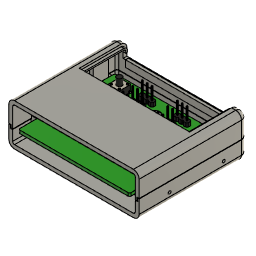
openC64case v22 (Autodesk Fusion 360 design; units mm, degrees)
Autodesk Fusion 360 part; units mm, degrees
(part 1 of 2)
sketch "Skizze1" plane through (0, 0, 0) normal (0, 0, 1) x (1, 0, 0)
  line L0 (44.1492, 35.54) -> (43.8162, 36.0162)
  line L1 (41.7212, 35.54) -> (41.7212, 36.54)
  line L2 (44.1492, 36.3495) -> (44.1492, 36.2067)
  line L3 (44.9592, 36.54) -> (45.0542, 36.4924)
  line L4 (42.5302, 36.54) -> (43.1972, 35.54)
  line L5 (42.5382, 48.2051) -> (42.4902, 48.3956)
  line L6 (43.5782, 35.54) -> (43.5782, 36.54)
  line L7 (42.4902, 48.7289) -> (42.5382, 48.9194)
  line L8 (43.5782, 36.54) -> (43.9592, 36.54)
  line L9 (42.1972, 35.54) -> (41.7212, 35.54)
  line L10 (44.7682, 36.54) -> (44.9592, 36.54)
  line L11 (43.1972, 36.54) -> (42.5302, 35.54)
  line L12 (45.6262, 36.54) -> (45.9592, 35.8257)
  line L13 (44.0542, 36.0638) -> (43.9592, 36.0162)
  line L14 (42.6332, 48.1098) -> (42.5382, 48.2051)
  line L15 (45.0542, 35.5876) -> (44.9592, 35.54)
  line L16 (42.2922, 41.0613) -> (42.1022, 41.0613)
  line L17 (44.5782, 36.3972) -> (44.6732, 36.4924)
  line L18 (45.1492, 35.6829) -> (45.0542, 35.5876)
  line L19 (45.1972, 35.8734) -> (45.1492, 35.6829)
  line L20 (42.6332, 49.0146) -> (42.7292, 49.0622)
  line L21 (44.9592, 35.54) -> (44.7682, 35.54)
  line L22 (45.0542, 36.4924) -> (45.1492, 36.3972)
  line L23 (43.9592, 36.54) -> (44.0542, 36.4924)
  line L24 (44.1492, 36.2067) -> (44.1022, 36.1114)
  line L25 (42.1492, 41.6327) -> (42.0062, 41.6327)
  line L26 (44.5782, 35.6829) -> (44.5302, 35.8734)
  line L27 (42.5382, 48.9194) -> (42.6332, 49.0146)
  line L28 (41.7212, 36.54) -> (42.1972, 36.54)
  line L29 (43.9592, 36.0162) -> (43.5782, 36.0162)
  line L30 (44.6732, 35.5876) -> (44.5782, 35.6829)
  line L31 (42.5782, 40.6327) -> (42.9112, 41.6327)
  line L32 (43.5782, 41.6327) -> (43.9112, 40.9184)
  line L33 (44.1022, 36.1114) -> (44.0542, 36.0638)
  line L34 (44.0542, 36.4924) -> (44.1022, 36.4448)
  line L35 (41.6732, 41.0613) -> (41.7212, 40.8708)
  line L36 (42.6732, 40.9184) -> (43.1492, 40.9184)
  line L37 (45.6262, 35.54) -> (45.6262, 36.54)
  line L38 (45.1492, 36.3972) -> (45.1972, 36.2067)
  line L39 (41.7212, 36.0638) -> (42.0542, 36.0638)
  line L40 (44.1972, 27.6866) -> (14.7332, 27.6866)
  line L41 (28.1952, 27.6866) -> (28.1952, 17.5266)
  line L42 (42.0062, 41.6327) -> (41.8642, 41.5851)
  line L43 (48.2612, 15.4946) -> (48.2612, 29.7186)
  line L44 (8.1452, 19.1706) -> (8.1452, 26.1706)
  line L45 (11.6852, 21.3366) -> (10.6692, 21.3366)
  line L46 (57.6592, 0.0006) -> (0.7632, 0.0006)
  line L47 (47.2452, 31.4966) -> (47.2452, 13.7166)
  line L48 (44.7212, 40.6327) -> (44.7212, 41.6327)
  line L49 (11.6852, 23.8766) -> (11.6852, 21.3366)
  line L50 (43.9112, 40.9184) -> (44.2452, 41.6327)
  line L51 (41.8642, 40.6803) -> (42.0062, 40.6327)
  line L52 (41.7212, 41.3946) -> (41.6732, 41.2041)
  line L53 (11.6852, 13.7166) -> (11.6852, 31.4966)
  line L54 (46.2922, 36.54) -> (46.2922, 35.54)
  line L55 (48.2612, 29.7186) -> (10.6692, 29.7186)
  line L56 (42.2452, 41.5851) -> (42.1492, 41.6327)
  line L57 (44.7212, 41.6327) -> (45.1972, 41.6327)
  line L58 (44.2452, 41.6327) -> (44.2452, 40.6327)
  line L59 (45.1972, 40.6327) -> (44.7212, 40.6327)
  line L60 (42.9112, 41.6327) -> (43.2452, 40.6327)
  line L61 (11.6852, 23.8766) -> (10.6692, 23.8766)
  line L62 (44.5302, 36.2067) -> (44.5782, 36.3972)
  arc A0 (12.9552, 22.6066) -> (11.6852, 23.8766) centre (11.6852, 22.6066) ccw
  line L63 (41.7682, 40.7756) -> (41.8642, 40.6803)
  line L64 (9.9952, 22.1706) -> (9.9952, 23.1706)
  line L65 (44.1972, 27.6866) -> (44.1972, 17.5266)
  line L66 (10.6692, 29.7186) -> (10.6692, 15.4946)
  line L67 (41.7212, 40.8708) -> (41.7682, 40.7756)
  line L68 (42.2922, 40.728) -> (42.2922, 41.0613)
  line L69 (41.8642, 41.5851) -> (41.7682, 41.4899)
  line L70 (44.5302, 35.8734) -> (44.5302, 36.2067)
  line L71 (42.0062, 40.6327) -> (42.1022, 40.6327)
  line L72 (41.7682, 41.4899) -> (41.7212, 41.3946)
  arc A1 (11.6852, 21.3366) -> (12.9552, 22.6066) centre (11.6852, 22.6066) ccw
  line L73 (44.6732, 36.4924) -> (44.7682, 36.54)
  line L74 (8.2952, 23.1706) -> (8.2952, 22.1706)
  line L75 (14.7332, 27.6866) -> (14.7332, 17.5266)
  line L76 (0.0012, 0.7626) -> (0.0012, 49.5306)
  line L77 (44.7682, 35.54) -> (44.6732, 35.5876)
  line L78 (45.9592, 35.8257) -> (46.2922, 36.54)
  line L79 (44.7212, 41.1565) -> (45.0542, 41.1565)
  line L80 (43.5782, 40.6327) -> (43.5782, 41.6327)
  line L81 (41.6732, 41.2041) -> (41.6732, 41.0613)
  line L82 (42.1022, 40.6327) -> (42.2452, 40.6803)
  line L83 (42.2452, 40.6803) -> (42.2922, 40.728)
  line L84 (1.2712, 50.8006) -> (57.1512, 50.8006)
  line L85 (11.6852, 31.4966) -> (47.2452, 31.4966)
  line L86 (58.4212, 49.5306) -> (58.4212, 0.7626)
  line L87 (8.1452, 19.1706) -> (10.1452, 19.1706)
  line L88 (9.9955, 48.1389) -> (9.8745, 48.1994)
  line L89 (7.0322, 48.8646) -> (7.516, 48.8646)
  line L90 (10.1164, 47.9575) -> (10.056, 48.0784)
  circle A2 centre (9.6024, 43.4702) radius 0.8032
  line L91 (7.516, 48.1994) -> (7.0322, 48.1994)
  line L92 (7.516, 48.8646) -> (7.6369, 48.8042)
  line L93 (7.6974, 48.7437) -> (7.7579, 48.6227)
  line L94 (8.3022, 47.5946) -> (8.3022, 48.8646)
  line L95 (7.0322, 47.5946) -> (7.0322, 48.8646)
  line L96 (7.6974, 48.3204) -> (7.6369, 48.2599)
  circle A3 centre (29.2112, 42.5006) radius 2.736
  circle A4 centre (39.8794, 46.2286) radius 0.961
  line L97 (9.935, 48.8646) -> (10.1164, 48.8042)
  line L98 (18.0606, 45.2126) -> (18.0606, 47.2446)
  circle A5 centre (21.4642, 46.2286) radius 0.9367
  line L99 (7.7579, 47.5946) -> (7.3345, 48.1994)
  line L100 (9.3907, 47.6551) -> (9.5722, 47.5946)
  line L101 (10.056, 48.0784) -> (9.9955, 48.1389)
  line L102 (10.1164, 47.8365) -> (10.1164, 47.9575)
  line L103 (14.7332, 17.5266) -> (44.1972, 17.5266)
  circle A6 centre (39.8791, 41.1486) radius 1.0208
  line L104 (9.3907, 48.6227) -> (9.4512, 48.7437)
  line L105 (7.6369, 48.8042) -> (7.6974, 48.7437)
  line L106 (11.6852, 13.7166) -> (47.2452, 13.7166)
  line L107 (7.7579, 48.4413) -> (7.6974, 48.3204)
  line L108 (7.6369, 48.2599) -> (7.516, 48.1994)
  line L109 (9.8745, 47.5946) -> (9.9955, 47.6551)
  line L110 (48.2612, 15.4946) -> (10.6692, 15.4946)
  line L111 (10.056, 47.7156) -> (10.1164, 47.8365)
  line L112 (8.9069, 47.5946) -> (8.3022, 47.5946)
  line L113 (10.1452, 26.1706) -> (8.1452, 26.1706)
  line L114 (18.0606, 47.2446) -> (19.7878, 47.2446)
  circle A7 centre (39.8791, 36.0686) radius 1.0208
  line L115 (9.3907, 48.5018) -> (9.3907, 48.6227)
  line L116 (10.1452, 26.1706) -> (10.1452, 19.1706)
  line L117 (30.7352, 17.5266) -> (30.7352, 27.6866)
  line L118 (8.3022, 48.8646) -> (8.9069, 48.8646)
  line L119 (9.6326, 48.2599) -> (9.5117, 48.3204)
  line L120 (9.5117, 48.3204) -> (9.4512, 48.3808)
  line L121 (9.5722, 47.5946) -> (9.8745, 47.5946)
  line L122 (7.7579, 48.6227) -> (7.7579, 48.4413)
  line L123 (9.9955, 47.6551) -> (10.056, 47.7156)
  line L124 (8.3022, 48.2599) -> (8.7255, 48.2599)
  line L125 (9.8745, 48.1994) -> (9.6326, 48.2599)
  line L126 (19.7878, 42.1646) -> (19.7878, 40.1326)
  line L127 (10.6607, 47.5946) -> (10.6607, 48.8646)
  circle A8 centre (21.4642, 36.0686) radius 0.9608
  line L128 (18.0606, 40.1326) -> (18.0606, 42.1646)
  line L129 (9.4512, 48.7437) -> (9.5117, 48.8042)
  line L130 (9.5117, 48.8042) -> (9.6326, 48.8646)
  line L131 (9.6326, 48.8646) -> (9.935, 48.8646)
  line L132 (36.3232, 37.0846) -> (38.3552, 37.0846)
  circle A9 centre (6.3512, 45.7206) radius 1.0043
  line L133 (19.7878, 45.2126) -> (18.0606, 45.2126)
  line L134 (19.7878, 47.2446) -> (19.7878, 45.2126)
  circle A10 centre (12.8536, 41.2198) radius 1.0043
  line L135 (36.4756, 47.2446) -> (38.2028, 47.2446)
  line L136 (38.3552, 37.0846) -> (38.3552, 35.0526)
  line L137 (19.7878, 37.0846) -> (19.7878, 35.0526)
  line L138 (18.0606, 37.0846) -> (19.7878, 37.0846)
  circle A11 centre (24.0042, 36.0686) radius 0.9608
  line L139 (9.4512, 48.3808) -> (9.3907, 48.5018)
  line L140 (38.2028, 47.2446) -> (38.2028, 45.2126)
  line L141 (11.2655, 47.5946) -> (10.6607, 47.5946)
  line L142 (36.3232, 40.1326) -> (36.3232, 42.1646)
  line L143 (38.2028, 45.2126) -> (36.4756, 45.2126)
  line L144 (18.0606, 42.1646) -> (19.7878, 42.1646)
  line L145 (10.6607, 48.2599) -> (11.0841, 48.2599)
  line L146 (36.3232, 42.1646) -> (38.3552, 42.1646)
  circle A12 centre (6.3512, 41.2198) radius 1.0043
  line L147 (38.3552, 42.1646) -> (38.3552, 40.1326)
  line L148 (18.0606, 35.0526) -> (18.0606, 37.0846)
  line L149 (36.3232, 35.0526) -> (36.3232, 37.0846)
  line L150 (38.3552, 35.0526) -> (36.3232, 35.0526)
  line L151 (19.7878, 35.0526) -> (18.0606, 35.0526)
  circle A13 centre (24.0042, 41.1486) radius 0.9367
  line L152 (11.9912, 47.5946) -> (11.9912, 48.8646)
  circle A14 centre (42.4192, 46.2286) radius 0.9612
  circle A15 centre (24.0042, 46.2286) radius 0.9608
  line L153 (10.6607, 48.8646) -> (11.2655, 48.8646)
  line L154 (36.4756, 45.2126) -> (36.4756, 47.2446)
  line L155 (19.7878, 40.1326) -> (18.0606, 40.1326)
  line L156 (38.3552, 40.1326) -> (36.3232, 40.1326)
  circle A16 centre (12.8536, 45.7206) radius 1.0043
  line L157 (11.6284, 48.8646) -> (12.3541, 48.8646)
  circle A17 centre (21.4642, 41.1486) radius 0.9099
  line L158 (41.7292, 48.0622) -> (41.7292, 49.0622)
  line L159 (42.2052, 48.0622) -> (41.7292, 48.0622)
  line L160 (18.3242, 48.586) -> (18.8956, 48.586)
  line L161 (43.1092, 48.9194) -> (43.1572, 48.7289)
  line L162 (43.0142, 49.0146) -> (43.1092, 48.9194)
  line L163 (36.8154, 48.586) -> (37.3868, 48.586)
  line L164 (43.1572, 48.3956) -> (43.1092, 48.2051)
  line L165 (24.2185, 49.0146) -> (24.3137, 49.0622)
  line L166 (43.1572, 48.7289) -> (43.1572, 48.3956)
  line L167 (19.3718, 48.0622) -> (19.3718, 49.0622)
  line L168 (42.9192, 48.0622) -> (42.7292, 48.0622)
  line L169 (42.7292, 48.0622) -> (42.6332, 48.1098)
  line L170 (24.7423, 48.3956) -> (24.6947, 48.2051)
  line L171 (24.1232, 48.9194) -> (24.2185, 49.0146)
  line L172 (24.5042, 48.0622) -> (24.3137, 48.0622)
  line L173 (42.9192, 49.0622) -> (43.0142, 49.0146)
  line L174 (36.8154, 48.0622) -> (36.8154, 49.0622)
  line L175 (37.863, 48.0622) -> (37.863, 49.0622)
  line L176 (42.7292, 49.0622) -> (42.9192, 49.0622)
  line L177 (43.1092, 48.2051) -> (43.0142, 48.1098)
  line L178 (43.0142, 48.1098) -> (42.9192, 48.0622)
  line L179 (24.7423, 48.7289) -> (24.7423, 48.3956)
  line L180 (45.1972, 36.2067) -> (45.1972, 35.8734)
  line L181 (42.4902, 48.3956) -> (42.4902, 48.7289)
  line L182 (44.1022, 36.4448) -> (44.1492, 36.3495)
  line L183 (24.5994, 48.1098) -> (24.5042, 48.0622)
  line L184 (12.6024, 46.2702) -> (12.6024, 44.9202)
  arc A18 (12.0524, 46.0202) -> (12.1024, 45.2702) centre (11.7522, 45.6235) ccw
  line L185 (6.1024, 45.3702) -> (6.6024, 45.3702)
  circle A19 centre (9.6024, 43.4702) radius 1.75
  line L186 (6.8524, 40.4702) -> (6.8024, 40.4702)
  arc A20 (12.0524, 40.9202) -> (12.0524, 41.7202) centre (11.7524, 41.3202) ccw
  circle A21 centre (9.6024, 43.4702) radius 1.4
  line L187 (6.6024, 46.0702) -> (6.1024, 46.0702)
  line L188 (12.6024, 42.0702) -> (12.6024, 40.6702)
  line L189 (12.3524, 46.4702) -> (12.4024, 46.4702)
  line L190 (6.6024, 44.9202) -> (6.6024, 46.2702)
  line L191 (12.0024, 40.4702) -> (6.8524, 40.4702)
  line L192 (12.4024, 40.4702) -> (12.0024, 40.4702)
  line L193 (6.6024, 42.0202) -> (6.6024, 44.9202)
  arc A22 (7.1023, 41.6702) -> (7.1523, 40.9202) centre (7.4526, 41.3169) ccw
  line L194 (6.6024, 45.3702) -> (6.6024, 46.0702)
  line L195 (6.1024, 46.0702) -> (6.1024, 45.3702)
  line L196 (12.6024, 44.9202) -> (12.6024, 42.0702)
  arc A23 (12.1024, 45.2702) -> (12.0524, 46.0202) centre (11.7522, 45.6235) ccw
  arc A24 (6.6024, 40.6702) -> (6.8024, 40.4702) centre (6.8024, 40.6702) ccw
  arc A25 (7.1523, 40.9202) -> (7.1023, 41.6702) centre (7.4526, 41.3169) ccw
  line L197 (6.8024, 46.4702) -> (6.8524, 46.4702)
  arc A26 (12.0524, 41.7202) -> (12.0524, 40.9202) centre (11.7524, 41.3202) ccw
  arc A27 (12.4024, 40.4702) -> (12.6024, 40.6702) centre (12.4024, 40.6702) ccw
  line L198 (6.8524, 46.4702) -> (12.3524, 46.4702)
  arc A28 (6.8024, 46.4702) -> (6.6024, 46.2702) centre (6.8024, 46.2702) ccw
  line L199 (6.6024, 40.8702) -> (6.6024, 41.5702)
  line L200 (20.1942, 46.8636) -> (20.5117, 47.1811)
  line L201 (20.8292, 47.4986) -> (22.0992, 47.4986)
  line L202 (19.8767, 45.2761) -> (19.5592, 44.9586)
  line L203 (20.8292, 47.4986) -> (22.0992, 47.4986)
  line L204 (19.5592, 44.9586) -> (17.6542, 44.9586)
  line L205 (22.4167, 47.1811) -> (22.7341, 46.8636)
  line L206 (23.0517, 47.1811) -> (23.3692, 47.4986)
  line L207 (17.6542, 46.8636) -> (17.6542, 45.5936)
  line L208 (20.1942, 46.8636) -> (20.1942, 45.5936)
  line L209 (12.6024, 40.8702) -> (13.1024, 40.8702)
  line L210 (12.6024, 46.0702) -> (12.6024, 45.3702)
  line L211 (12.6024, 41.5702) -> (12.6024, 40.8702)
  line L212 (22.7341, 46.8636) -> (22.7341, 45.5936)
  line L213 (22.0992, 47.4986) -> (22.4167, 47.1811)
  line L214 (20.5117, 45.2761) -> (20.1942, 45.5936)
  line L215 (18.2891, 47.4986) -> (19.5592, 47.4986)
  line L216 (6.1024, 41.5702) -> (6.1024, 40.8702)
  line L217 (22.7341, 46.8636) -> (23.0517, 47.1811)
  line L218 (13.1024, 45.3702) -> (13.1024, 46.0702)
  arc A29 (12.6024, 46.2702) -> (12.4024, 46.4702) centre (12.4024, 46.2702) ccw
  line L219 (6.6024, 40.6702) -> (6.6024, 42.0202)
  arc A30 (7.1523, 45.2202) -> (7.1023, 45.9702) centre (7.4526, 45.6169) ccw
  arc A31 (7.1023, 45.9702) -> (7.1523, 45.2202) centre (7.4526, 45.6169) ccw
  line L220 (20.1942, 45.5936) -> (19.8767, 45.2761)
  line L221 (6.6024, 41.5702) -> (6.1024, 41.5702)
  line L222 (22.0992, 44.9586) -> (20.8292, 44.9586)
  line L223 (18.2891, 47.4986) -> (17.6542, 46.8636)
  line L224 (13.1024, 40.8702) -> (13.1024, 41.5702)
  line L225 (13.1024, 46.0702) -> (12.6024, 46.0702)
  line L226 (19.5592, 47.4986) -> (19.8767, 47.1811)
  line L227 (19.8767, 47.1811) -> (20.1942, 46.8636)
  line L228 (12.6024, 45.3702) -> (13.1024, 45.3702)
  line L229 (17.6542, 45.5936) -> (17.6542, 44.9586)
  line L230 (6.1024, 40.8702) -> (6.6024, 40.8702)
  line L231 (21.7182, 46.4826) -> (21.2102, 46.4826)
  line L232 (19.1782, 45.9746) -> (19.1782, 46.4826)
  line L233 (19.8767, 40.1961) -> (19.5592, 39.8786)
  line L234 (24.6392, 47.4986) -> (25.2742, 46.8636)
  line L235 (20.8292, 44.9586) -> (20.5117, 45.2761)
  line L236 (18.2891, 42.4186) -> (17.6542, 41.7836)
  line L237 (17.6542, 41.7836) -> (17.6542, 40.5136)
  line L238 (20.5117, 42.1011) -> (20.8292, 42.4186)
  line L239 (20.5117, 47.1811) -> (20.8292, 47.4986)
  line L240 (20.8292, 42.4186) -> (22.0992, 42.4186)
  line L241 (25.2742, 46.8636) -> (25.2742, 45.5936)
  line L242 (22.7341, 45.5936) -> (22.4167, 45.2761)
  line L243 (21.2102, 45.9746) -> (21.7182, 45.9746)
  line L244 (20.1942, 40.5136) -> (19.8767, 40.1961)
  line L245 (17.6542, 40.5136) -> (17.6542, 39.8786)
  line L246 (19.5592, 42.4186) -> (19.8767, 42.1011)
  line L247 (19.5592, 39.8786) -> (17.6542, 39.8786)
  line L248 (24.2582, 46.4826) -> (23.7502, 46.4826)
  line L249 (19.1782, 46.4826) -> (18.6702, 46.4826)
  line L250 (18.6702, 46.4826) -> (18.6702, 45.9746)
  line L251 (25.2742, 45.5936) -> (24.6392, 44.9586)
  line L252 (23.0517, 45.2761) -> (22.7341, 45.5936)
  line L253 (21.2102, 46.4826) -> (21.2102, 45.9746)
  line L254 (22.0992, 39.8786) -> (20.8292, 39.8786)
  line L255 (13.1024, 41.5702) -> (12.6024, 41.5702)
  line L256 (21.7182, 45.9746) -> (21.7182, 46.4826)
  line L257 (23.3692, 44.9586) -> (23.0517, 45.2761)
  line L258 (20.5117, 40.1961) -> (20.1942, 40.5136)
  line L259 (24.6392, 44.9586) -> (23.3692, 44.9586)
  line L260 (18.6702, 45.9746) -> (19.1782, 45.9746)
  line L261 (20.1942, 41.7836) -> (20.5117, 42.1011)
  line L262 (23.7502, 45.9746) -> (24.2582, 45.9746)
  line L263 (22.4167, 45.2761) -> (22.0992, 44.9586)
  line L264 (18.2891, 42.4186) -> (19.5592, 42.4186)
  line L265 (20.8292, 39.8786) -> (20.5117, 40.1961)
  line L266 (19.8767, 42.1011) -> (20.1942, 41.7836)
  line L267 (20.1942, 41.7836) -> (20.1942, 40.5136)
  line L268 (23.3692, 47.4986) -> (24.6392, 47.4986)
  line L269 (24.2582, 41.4026) -> (23.7502, 41.4026)
  line L270 (23.7502, 46.4826) -> (23.7502, 45.9746)
  line L271 (18.6702, 40.8946) -> (19.1782, 40.8946)
  line L272 (23.7502, 40.8946) -> (24.2582, 40.8946)
  line L273 (22.4167, 40.1961) -> (22.0992, 39.8786)
  line L274 (24.2582, 45.9746) -> (24.2582, 46.4826)
  line L275 (19.1782, 40.8946) -> (19.1782, 41.4026)
  line L276 (23.7502, 41.4026) -> (23.7502, 40.8946)
  line L277 (20.1942, 36.7036) -> (20.1942, 35.4336)
  line L278 (21.7182, 36.3226) -> (21.2102, 36.3226)
  line L279 (23.3692, 42.4186) -> (24.6392, 42.4186)
  line L280 (25.2742, 41.7836) -> (25.2742, 40.5136)
  line L281 (21.2102, 36.3226) -> (21.2102, 35.8146)
  line L282 (22.7341, 36.7036) -> (22.7341, 35.4336)
  line L283 (22.7341, 35.4336) -> (22.4167, 35.1161)
  line L284 (17.6542, 36.7036) -> (17.6542, 35.4336)
  line L285 (24.6392, 39.8786) -> (23.3692, 39.8786)
  line L286 (19.8767, 37.0211) -> (20.1942, 36.7036)
  line L287 (20.1942, 35.4336) -> (19.8767, 35.1161)
  line L288 (23.0517, 35.1161) -> (22.7341, 35.4336)
  line L289 (24.6392, 34.7986) -> (23.3692, 34.7986)
  line L290 (23.3692, 34.7986) -> (23.0517, 35.1161)
  line L291 (19.1782, 35.8146) -> (19.1782, 36.3226)
  line L292 (19.5592, 34.7986) -> (17.6542, 34.7986)
  line L293 (20.5117, 37.0211) -> (20.8292, 37.3386)
  line L294 (21.7182, 40.8946) -> (21.7182, 41.4026)
  line L295 (22.0992, 42.4186) -> (22.4167, 42.1011)
  line L296 (23.0517, 40.1961) -> (22.7341, 40.5136)
  line L297 (21.2102, 41.4026) -> (21.2102, 40.8946)
  line L298 (18.2891, 37.3386) -> (17.6542, 36.7036)
  line L299 (21.2102, 40.8946) -> (21.7182, 40.8946)
  line L300 (25.2742, 35.4336) -> (24.6392, 34.7986)
  line L301 (24.2582, 35.8146) -> (24.2582, 36.3226)
  line L302 (18.2891, 37.3386) -> (19.5592, 37.3386)
  line L303 (19.8767, 35.1161) -> (19.5592, 34.7986)
  line L304 (22.7341, 40.5136) -> (22.4167, 40.1961)
  line L305 (21.7182, 41.4026) -> (21.2102, 41.4026)
  line L306 (22.4167, 42.1011) -> (22.7341, 41.7836)
  line L307 (25.2742, 40.5136) -> (24.6392, 39.8786)
  line L308 (20.8292, 42.4186) -> (22.0992, 42.4186)
  line L309 (24.2582, 36.3226) -> (23.7502, 36.3226)
  line L310 (22.0992, 34.7986) -> (20.8292, 34.7986)
  line L311 (20.8292, 34.7986) -> (20.5117, 35.1161)
  line L312 (22.0992, 37.3386) -> (22.4167, 37.0211)
  line L313 (17.6542, 35.4336) -> (17.6542, 34.7986)
  line L314 (23.0517, 37.0211) -> (23.3692, 37.3386)
  line L315 (22.7341, 41.7836) -> (22.7341, 40.5136)
  line L316 (18.6702, 41.4026) -> (18.6702, 40.8946)
  line L317 (22.7341, 41.7836) -> (23.0517, 42.1011)
  line L318 (19.1782, 41.4026) -> (18.6702, 41.4026)
  line L319 (19.5592, 37.3386) -> (19.8767, 37.0211)
  line L320 (23.7502, 35.8146) -> (24.2582, 35.8146)
  line L321 (24.6392, 42.4186) -> (25.2742, 41.7836)
  line L322 (23.0517, 42.1011) -> (23.3692, 42.4186)
  line L323 (24.2582, 40.8946) -> (24.2582, 41.4026)
  line L324 (21.7182, 35.8146) -> (21.7182, 36.3226)
  line L325 (23.3692, 39.8786) -> (23.0517, 40.1961)
  line L326 (43.6894, 46.8636) -> (43.6894, 45.5936)
  line L327 (20.8292, 37.3386) -> (22.0992, 37.3386)
  line L328 (23.3692, 37.3386) -> (24.6392, 37.3386)
  line L329 (40.5144, 44.9586) -> (39.2444, 44.9586)
  line L330 (20.8292, 37.3386) -> (22.0992, 37.3386)
  line L331 (36.7043, 47.4986) -> (37.9744, 47.4986)
  line L332 (36.0694, 46.8636) -> (36.0694, 45.5936)
  line L333 (40.5144, 47.4986) -> (40.8319, 47.1811)
  line L334 (37.9744, 47.4986) -> (38.2919, 47.1811)
  line L335 (38.9269, 45.2761) -> (38.6094, 45.5936)
  line L336 (41.1493, 46.8636) -> (41.4669, 47.1811)
  line L337 (41.4669, 47.1811) -> (41.7844, 47.4986)
  line L338 (41.1493, 45.5936) -> (40.8319, 45.2761)
  line L339 (24.6392, 37.3386) -> (25.2742, 36.7036)
  line L340 (21.2102, 35.8146) -> (21.7182, 35.8146)
  line L341 (22.4167, 37.0211) -> (22.7341, 36.7036)
  line L342 (38.9269, 47.1811) -> (39.2444, 47.4986)
  line L343 (38.6094, 46.8636) -> (38.9269, 47.1811)
  line L344 (23.7502, 36.3226) -> (23.7502, 35.8146)
  line L345 (39.2444, 47.4986) -> (40.5144, 47.4986)
  line L346 (41.7844, 47.4986) -> (43.0544, 47.4986)
  line L347 (25.2742, 36.7036) -> (25.2742, 35.4336)
  line L348 (40.8319, 45.2761) -> (40.5144, 44.9586)
  line L349 (43.0544, 47.4986) -> (43.6894, 46.8636)
  line L350 (22.4167, 35.1161) -> (22.0992, 34.7986)
  line L351 (18.6702, 35.8146) -> (19.1782, 35.8146)
  line L352 (18.6702, 36.3226) -> (18.6702, 35.8146)
  line L353 (36.0694, 45.5936) -> (36.0694, 44.9586)
  line L354 (39.2444, 47.4986) -> (40.5144, 47.4986)
  line L355 (39.2444, 44.9586) -> (38.9269, 45.2761)
  line L356 (43.6894, 45.5936) -> (43.0544, 44.9586)
  line L357 (41.4669, 45.2761) -> (41.1493, 45.5936)
  line L358 (41.7844, 44.9586) -> (41.4669, 45.2761)
  line L359 (37.9744, 44.9586) -> (36.0694, 44.9586)
  line L360 (38.2919, 47.1811) -> (38.6094, 46.8636)
  line L361 (40.8319, 47.1811) -> (41.1493, 46.8636)
  line L362 (20.1942, 36.7036) -> (20.5117, 37.0211)
  line L363 (38.2919, 45.2761) -> (37.9744, 44.9586)
  line L364 (38.6094, 46.8636) -> (38.6094, 45.5936)
  line L365 (43.0544, 44.9586) -> (41.7844, 44.9586)
  line L366 (38.6094, 45.5936) -> (38.2919, 45.2761)
  line L367 (20.5117, 35.1161) -> (20.1942, 35.4336)
  line L368 (36.7043, 47.4986) -> (36.0694, 46.8636)
  line L369 (22.7341, 36.7036) -> (23.0517, 37.0211)
  line L370 (19.1782, 36.3226) -> (18.6702, 36.3226)
  line L371 (41.1493, 46.8636) -> (41.1493, 45.5936)
  line L372 (40.1334, 46.4826) -> (39.6254, 46.4826)
  line L373 (37.5934, 45.9746) -> (37.5934, 46.4826)
  line L374 (37.0854, 46.4826) -> (37.0854, 45.9746)
  line L375 (41.149, 40.5136) -> (40.8316, 40.1961)
  line L376 (36.704, 37.3386) -> (37.9741, 37.3386)
  line L377 (36.704, 37.3386) -> (36.0691, 36.7036)
  line L378 (40.1331, 35.8146) -> (40.1331, 36.3226)
  line L379 (42.1654, 45.9746) -> (42.6734, 45.9746)
  line L380 (38.6091, 41.7836) -> (38.6091, 40.5136)
  line L381 (37.0851, 40.8946) -> (37.5931, 40.8946)
  line L382 (38.9266, 40.1961) -> (38.6091, 40.5136)
  line L383 (36.0691, 40.5136) -> (36.0691, 39.8786)
  line L384 (38.2916, 40.1961) -> (37.9741, 39.8786)
  line L385 (37.5931, 41.4026) -> (37.0851, 41.4026)
  line L386 (42.1654, 46.4826) -> (42.1654, 45.9746)
  line L387 (38.6091, 35.4336) -> (38.2916, 35.1161)
  line L388 (36.704, 42.4186) -> (37.9741, 42.4186)
  line L389 (40.8316, 40.1961) -> (40.5141, 39.8786)
  line L390 (39.2441, 42.4186) -> (40.5141, 42.4186)
  line L391 (40.5141, 39.8786) -> (39.2441, 39.8786)
  line L392 (40.1334, 45.9746) -> (40.1334, 46.4826)
  line L393 (42.6734, 46.4826) -> (42.1654, 46.4826)
  line L394 (37.0851, 41.4026) -> (37.0851, 40.8946)
  line L395 (38.6091, 40.5136) -> (38.2916, 40.1961)
  line L396 (41.149, 41.7836) -> (41.149, 40.5136)
  line L397 (38.2916, 42.1011) -> (38.6091, 41.7836)
  line L398 (39.6254, 46.4826) -> (39.6254, 45.9746)
  line L399 (37.0854, 45.9746) -> (37.5934, 45.9746)
  line L400 (39.2441, 39.8786) -> (38.9266, 40.1961)
  line L401 (39.2441, 42.4186) -> (40.5141, 42.4186)
  line L402 (39.6254, 45.9746) -> (40.1334, 45.9746)
  line L403 (42.6734, 45.9746) -> (42.6734, 46.4826)
  line L404 (37.0851, 36.3226) -> (37.0851, 35.8146)
  line L405 (40.8316, 35.1161) -> (40.5141, 34.7986)
  line L406 (40.5141, 42.4186) -> (40.8316, 42.1011)
  line L407 (40.5141, 34.7986) -> (39.2441, 34.7986)
  line L408 (38.2916, 37.0211) -> (38.6091, 36.7036)
  line L409 (36.704, 42.4186) -> (36.0691, 41.7836)
  line L410 (37.9741, 42.4186) -> (38.2916, 42.1011)
  line L411 (40.8316, 42.1011) -> (41.149, 41.7836)
  line L412 (37.9741, 39.8786) -> (36.0691, 39.8786)
  line L413 (37.0851, 35.8146) -> (37.5931, 35.8146)
  line L414 (39.2441, 37.3386) -> (40.5141, 37.3386)
  line L415 (38.9266, 42.1011) -> (39.2441, 42.4186)
  line L416 (36.0691, 41.7836) -> (36.0691, 40.5136)
  line L417 (41.149, 36.7036) -> (41.149, 35.4336)
  line L418 (40.1331, 36.3226) -> (39.6251, 36.3226)
  line L419 (37.5934, 46.4826) -> (37.0854, 46.4826)
  line L420 (38.6091, 41.7836) -> (38.9266, 42.1011)
  line L421 (45.3002, 45.6492) -> (45.2052, 45.6968)
  line L422 (45.2052, 45.6968) -> (45.1102, 45.7921)
  line L423 (45.1102, 45.7921) -> (45.0622, 45.9826)
  line L424 (46.1572, 45.6492) -> (46.1572, 46.6492)
  line L425 (39.6251, 36.3226) -> (39.6251, 35.8146)
  line L426 (39.2441, 37.3386) -> (40.5141, 37.3386)
  line L427 (40.8316, 37.0211) -> (41.149, 36.7036)
  line L428 (38.9266, 37.0211) -> (39.2441, 37.3386)
  line L429 (39.2441, 34.7986) -> (38.9266, 35.1161)
  line L430 (38.6091, 36.7036) -> (38.6091, 35.4336)
  line L431 (37.9741, 37.3386) -> (38.2916, 37.0211)
  line L432 (40.1331, 40.8946) -> (40.1331, 41.4026)
  line L433 (36.0691, 36.7036) -> (36.0691, 35.4336)
  line L434 (37.5931, 36.3226) -> (37.0851, 36.3226)
  line L435 (45.0622, 45.9826) -> (45.0622, 46.3159)
  arc A32 (1.2712, 50.8006) -> (0.0012, 49.5306) centre (1.2712, 49.5306) ccw
  line L436 (44.6812, 46.4587) -> (44.6812, 46.3159)
  line L437 (39.6251, 35.8146) -> (40.1331, 35.8146)
  line L438 (39.6251, 40.8946) -> (40.1331, 40.8946)
  line L439 (44.6812, 46.3159) -> (44.6342, 46.2206)
  line L440 (36.0691, 35.4336) -> (36.0691, 34.7986)
  line L441 (41.149, 35.4336) -> (40.8316, 35.1161)
  line L442 (45.4912, 46.6492) -> (45.5862, 46.6016)
  line L443 (40.1331, 41.4026) -> (39.6251, 41.4026)
  line L444 (38.2916, 35.1161) -> (37.9741, 34.7986)
  line L445 (38.6091, 36.7036) -> (38.9266, 37.0211)
  line L446 (38.9266, 35.1161) -> (38.6091, 35.4336)
  line L447 (37.9741, 34.7986) -> (36.0691, 34.7986)
  line L448 (37.5931, 40.8946) -> (37.5931, 41.4026)
  line L449 (37.5931, 35.8146) -> (37.5931, 36.3226)
  line L450 (40.5141, 37.3386) -> (40.8316, 37.0211)
  line L451 (39.6251, 41.4026) -> (39.6251, 40.8946)
  line L452 (45.2052, 46.6016) -> (45.3002, 46.6492)
  line L453 (44.1102, 45.6492) -> (44.1102, 46.6492)
  line L454 (44.1102, 46.6492) -> (44.4912, 46.6492)
  line L455 (44.5862, 46.6016) -> (44.6342, 46.554)
  line L456 (45.5862, 46.6016) -> (45.6812, 46.5064)
  line L457 (44.6812, 45.6492) -> (44.3482, 46.1254)
  line L458 (44.4912, 46.1254) -> (44.1102, 46.1254)
  line L459 (45.5862, 45.6968) -> (45.4912, 45.6492)
  arc A33 (0.0012, 0.7626) -> (0.7632, 0.0006) centre (0.7632, 0.7626) ccw
  line L460 (15.0667, 40.9819) -> (15.5429, 40.9819)
  line L461 (16.9715, 35.6162) -> (16.8762, 35.6638)
  line L462 (16.8762, 35.6638) -> (16.8286, 35.7115)
  line L463 (17.4001, 35.7115) -> (17.3524, 35.6638)
  line L464 (45.1102, 46.5064) -> (45.2052, 46.6016)
  line L465 (16.2096, 36.6162) -> (16.1143, 36.4734)
  arc A34 (57.6592, 0.0006) -> (58.4212, 0.7626) centre (57.6592, 0.7626) ccw
  line L466 (15.3048, 41.6962) -> (15.6382, 40.6962)
  line L467 (16.0191, 36.3781) -> (15.9239, 36.3305)
  line L468 (17.4001, 36.14) -> (17.4477, 36.0448)
  line L469 (17.4477, 36.6162) -> (17.1143, 36.2353)
  line L470 (46.8242, 46.6492) -> (46.8242, 45.6492)
  line L471 (44.6342, 46.2206) -> (44.5862, 46.173)
  line L472 (15.3048, 36.6162) -> (15.6382, 35.6162)
  line L473 (16.2096, 40.6962) -> (16.2096, 41.6962)
  line L474 (17.4477, 35.8067) -> (17.4001, 35.7115)
  line L475 (46.4912, 45.9349) -> (46.8242, 46.6492)
  line L476 (17.2572, 35.6162) -> (16.9715, 35.6162)
  arc A35 (58.4212, 49.5306) -> (57.1512, 50.8006) centre (57.1512, 49.5306) ccw
  line L477 (14.9715, 35.6162) -> (15.3048, 36.6162)
  line L478 (44.5862, 46.173) -> (44.4912, 46.1254)
  line L479 (45.0622, 46.3159) -> (45.1102, 46.5064)
  line L480 (45.4912, 45.6492) -> (45.3002, 45.6492)
  line L481 (16.2096, 41.6962) -> (16.1143, 41.5534)
  line L482 (16.4953, 35.6162) -> (15.9239, 35.6162)
  line L483 (44.4912, 46.6492) -> (44.5862, 46.6016)
  line L484 (15.0667, 35.9019) -> (15.5429, 35.9019)
  line L485 (44.6342, 46.554) -> (44.6812, 46.4587)
  line L486 (45.7292, 46.3159) -> (45.7292, 45.9826)
  line L487 (16.0191, 41.4581) -> (15.9239, 41.4105)
  line L488 (16.2096, 35.6162) -> (16.2096, 36.6162)
  line L489 (16.8286, 36.6162) -> (17.4477, 36.6162)
  line L490 (46.1572, 46.6492) -> (46.4912, 45.9349)
  line L491 (45.6812, 46.5064) -> (45.7292, 46.3159)
  line L492 (17.3524, 36.1876) -> (17.4001, 36.14)
  line L493 (45.6812, 45.7921) -> (45.5862, 45.6968)
  line L494 (17.1143, 36.2353) -> (17.2572, 36.2353)
  line L495 (45.3002, 46.6492) -> (45.4912, 46.6492)
  line L496 (17.4477, 36.0448) -> (17.4477, 35.8067)
  line L497 (14.9715, 40.6962) -> (15.3048, 41.6962)
  line L498 (16.4953, 40.6962) -> (15.9239, 40.6962)
  line L499 (16.1143, 41.5534) -> (16.0191, 41.4581)
  line L500 (17.2572, 36.2353) -> (17.3524, 36.1876)
  line L501 (45.7292, 45.9826) -> (45.6812, 45.7921)
  line L502 (16.1143, 36.4734) -> (16.0191, 36.3781)
  line L503 (17.0191, 45.7762) -> (16.9239, 45.8238)
  line L504 (16.9239, 46.3476) -> (17.0191, 46.3953)
  line L505 (17.4001, 46.7762) -> (16.9239, 46.7762)
  line L506 (16.9239, 45.8238) -> (16.8762, 45.8715)
  line L507 (16.8762, 41.0296) -> (17.4953, 41.0296)
  line L508 (16.2096, 46.7762) -> (16.1143, 46.6334)
  line L509 (23.3137, 48.0622) -> (23.3137, 49.0622)
  line L510 (17.3524, 41.3629) -> (17.3524, 40.6962)
  line L511 (17.2572, 45.7762) -> (17.0191, 45.7762)
  line L512 (24.0756, 48.3956) -> (24.0756, 48.7289)
  line L513 (15.0667, 46.0619) -> (15.5429, 46.0619)
  line L514 (24.3137, 48.0622) -> (24.2185, 48.1098)
  line L515 (18.3242, 48.0622) -> (18.3242, 49.0622)
  line L516 (18.8956, 48.0622) -> (18.8956, 49.0622)
  line L517 (37.3868, 48.0622) -> (37.3868, 49.0622)
  line L518 (24.5994, 49.0146) -> (24.6947, 48.9194)
  line L519 (24.6947, 48.2051) -> (24.5994, 48.1098)
  line L520 (24.2185, 48.1098) -> (24.1232, 48.2051)
  line L521 (24.1232, 48.2051) -> (24.0756, 48.3956)
  line L522 (16.2096, 45.7762) -> (16.2096, 46.7762)
  line L523 (17.3524, 35.6638) -> (17.2572, 35.6162)
  line L524 (17.4477, 45.9667) -> (17.4001, 45.8715)
  line L525 (17.4001, 45.8715) -> (17.3524, 45.8238)
  line L526 (16.8762, 46.3) -> (16.9239, 46.3476)
  line L527 (24.6947, 48.9194) -> (24.7423, 48.7289)
  line L528 (23.7899, 48.0622) -> (23.3137, 48.0622)
  line L529 (17.1143, 41.7438) -> (16.8762, 41.0296)
  line L530 (16.0191, 46.5381) -> (15.9239, 46.4905)
  line L531 (17.3524, 46.3476) -> (17.4001, 46.3)
  line L532 (16.9239, 46.7762) -> (16.8762, 46.3)
  line L533 (15.3048, 46.7762) -> (15.6382, 45.7762)
  line L534 (16.1143, 46.6334) -> (16.0191, 46.5381)
  line L535 (17.4001, 46.3) -> (17.4477, 46.2048)
  line L536 (17.0191, 46.3953) -> (17.2572, 46.3953)
  line L537 (14.9715, 45.7762) -> (15.3048, 46.7762)
  line L538 (17.2572, 46.3953) -> (17.3524, 46.3476)
  line L539 (17.3524, 45.8238) -> (17.2572, 45.7762)
  line L540 (17.4477, 46.2048) -> (17.4477, 45.9667)
  line L541 (24.3137, 49.0622) -> (24.5042, 49.0622)
  line L542 (24.5042, 49.0622) -> (24.5994, 49.0146)
  line L543 (16.4953, 45.7762) -> (15.9239, 45.7762)
  line L544 (24.0756, 48.7289) -> (24.1232, 48.9194)
extrude "Extrusion1" add sketch "Skizze1" against normal blind 1.6 contours L2 L6 L8 L13 L23 L24 L29 L33 L34 L182 | L3 L10 L15 L17 L18 L19 L21 L22 L26 L30 L38 L62 L70 L73 L77 L180 | L5 L7 L14 L20 L27 L161 L162 L164 L166 L168 L169 L173 L176 L177 L178 L181 | L31 L36 L60 | L40 L65 L103 L117 | L40 L41 L103 L117 | L40 L41 L75 L103 | L43 L47 L55 L110 | L47 L53 L55 A0 A1 L110 | L47 L53 L106 L110 | L47 L53 L55 L85 | L45 L53 L66 L110 | L53 L55 L61 L66 | L45 L49 L53 L61 L66 | L49 L53 A0 A1 | L44 L87 L113 L116 | L46 L76 L84 L86 A32 A33 A34 A35 | L89 L91 L92 L93 L95 L96 L105 L107 L108 L122 | A2 | A4 | L98 L114 L133 L134 | A5 | A6 | A7 | L126 L128 L144 L155 | A8 | L132 L149 L377 | L132 L376 L377 L431 | L132 L136 L149 L150 L377 L387 L408 L431 L444 | L149 L150 L377 L433 L440 L444 L447 | L132 L136 L408 L431 | L136 L150 L387 L444 | L136 L387 L408 L430 | L405 L407 L414 L417 L426 L427 L428 L429 L430 L441 L445 L446 L450 | A9 A30 A31 | A9 A30 | A9 L190 L193 L194 L197 L198 A28 A30 A31 | A9 A10 A12 A16 A18 L191 L192 L193 L196 A25 A26 L198 A30 | A9 L185 L187 L190 L193 L195 L197 L198 A28 | A16 L184 A18 L189 L196 A23 L198 L210 A29 | A16 L184 L189 L196 L198 L218 A29 L225 L228 | A12 L186 L191 L193 A24 L216 L219 L221 L230 | A12 L186 L191 L193 A22 A24 A25 L199 L219 | A16 A18 A23 | A16 A18 | A12 A25 | A12 A22 A25 | L185 L187 L190 L194 L195 | L199 L216 L219 L221 L230 | A10 A20 L188 L192 L196 A26 A27 L211 | A10 L188 L192 L196 A27 L209 L224 L255 | L184 L210 L218 L225 L228 | A10 A20 A26 | A10 A26 | L188 L209 L211 L224 L255 | L135 L140 L143 L154 | L137 L138 L148 L151 | A11 | L142 L156 L383 L384 L409 L412 L416 | L142 L146 L147 L156 L384 L395 L397 L409 L410 | L142 L146 L409 | L147 L156 L384 L395 | L146 L388 L409 L410 | L146 L147 L397 L410 | L147 L380 L395 L397 | L375 L380 L382 L389 L390 L391 L396 L400 L401 L406 L411 L415 L420 | A13 | A14 | A15 | A17 | L165 L170 L171 L172 L179 L183 L512 L514 L518 L519 L520 L521 L527 L541 L542 L544 | A19 | A21 | L200 L201 L203 L205 L208 L212 L213 L214 L222 L235 L239 L242 L263 | L202 L204 L207 L208 L215 L220 L223 L226 L227 L229 | L206 L212 L217 L234 L241 L251 L252 L257 L259 L268 | L231 L243 L253 L256 | L232 L249 L250 L260 | L233 L236 L237 L244 L245 L246 L247 L264 L266 L267 | L238 L240 L254 L258 L261 L265 L267 L273 L295 L304 L306 L308 L315 | L279 L280 L285 L296 L307 L315 L317 L321 L322 L325 | L248 L262 L270 L274 | L269 L272 L276 L323 | L271 L275 L316 L318 | L277 L282 L283 L293 L310 L311 L312 L327 L330 L341 L350 L362 L367 | L277 L284 L286 L287 L292 L298 L302 L303 L313 L319 | L282 L288 L289 L290 L300 L314 L328 L339 L347 L369 | L278 L281 L324 L340 | L291 L351 L352 L370 | L294 L297 L299 L305 | L301 L309 L320 L344 | L326 L336 L337 L346 L349 L356 L357 L358 L365 L371 | L329 L333 L335 L338 L342 L343 L345 L348 L354 L355 L361 L364 L371 | L331 L332 L334 L353 L359 L360 L363 L364 L366 L368 | L372 L392 L398 L402 | L373 L374 L399 L419 | L378 L418 L425 L437 | L379 L386 L393 L403 | L381 L385 L394 L448 | L404 L413 L434 L449 | L421 L422 L423 L435 L442 L452 L456 L459 L464 L479 L480 L486 L491 L493 L495 L501 | L432 L438 L443 L451 | L436 L439 L453 L454 L455 L458 L471 L478 L483 L485 | L460 L466 L497 | L472 L477 L484 | L513 L533 L537 makes body 1
extrude "Extrusion2" add sketch "Skizze1" along normal blind 4.5 contours L40 L41 L103 L117 | L47 L53 L55 A0 A1 L110 | L47 L53 L106 L110 | L47 L53 L55 L85 bodies 1
extrude "Extrusion3" add sketch "Skizze1" along normal blind 3.5 contours A2 | A9 A30 A31 | A9 A30 | A9 L190 L193 L194 L197 L198 A28 A30 A31 | A9 A10 A12 A16 A18 L191 L192 L193 L196 A25 A26 L198 A30 | A16 L184 A18 L189 L196 A23 L198 L210 A29 | A12 L186 L191 L193 A22 A24 A25 L199 L219 | A16 A18 A23 | A16 A18 | A12 A25 | A12 A22 A25 | A10 A20 L188 L192 L196 A26 A27 L211 | A10 A20 A26 | A10 A26 | A19 | A21 bodies 1
extrude "Extrusion4" add sketch "Skizze1" along normal blind 2 contours A4 | L98 L114 L133 L134 | A5 | A6 | A7 | L126 L128 L144 L155 | A8 | L132 L376 L377 L431 | L132 L136 L149 L150 L377 L387 L408 L431 L444 | L149 L150 L377 L433 L440 L444 L447 | L136 L387 L408 L430 | L405 L407 L414 L417 L426 L427 L428 L429 L430 L441 L445 L446 L450 | L135 L140 L143 L154 | L137 L138 L148 L151 | A11 | L142 L156 L383 L384 L409 L412 L416 | L142 L146 L147 L156 L384 L395 L397 L409 L410 | L146 L388 L409 L410 | L147 L380 L395 L397 | L375 L380 L382 L389 L390 L391 L396 L400 L401 L406 L411 L415 L420 | A13 | A14 | A15 | A17 | L200 L201 L203 L205 L208 L212 L213 L214 L222 L235 L239 L242 L263 | L202 L204 L207 L208 L215 L220 L223 L226 L227 L229 | L206 L212 L217 L234 L241 L251 L252 L257 L259 L268 | L233 L236 L237 L244 L245 L246 L247 L264 L266 L267 | L238 L240 L254 L258 L261 L265 L267 L273 L295 L304 L306 L308 L315 | L279 L280 L285 L296 L307 L315 L317 L321 L322 L325 | L277 L282 L283 L293 L310 L311 L312 L327 L330 L341 L350 L362 L367 | L277 L284 L286 L287 L292 L298 L302 L303 L313 L319 | L282 L288 L289 L290 L300 L314 L328 L339 L347 L369 | L326 L336 L337 L346 L349 L356 L357 L358 L365 L371 | L329 L333 L335 L338 L342 L343 L345 L348 L354 L355 L361 L364 L371 | L331 L332 L334 L353 L359 L360 L363 L364 L366 L368 bodies 1
extrude "Extrusion5" add sketch "Skizze1" along normal blind 5 contours L44 L87 L113 L116 bodies 1
extrude "Extrusion6" add sketch "Skizze1" along normal blind 9.5 contours L40 L65 L103 L117 | L40 L41 L103 L117 | L40 L41 L75 L103 | L43 L47 L55 L110 | L47 L53 L55 A0 A1 L110 | L45 L53 L66 L110 | L53 L55 L61 L66 | L49 L53 A0 A1 bodies 1
extrude "Extrusion7" add sketch "Skizze1" along normal blind 7 separate body contours A2 | A21 makes body 2
extrude "Extrusion8" add sketch "Skizze1" along normal blind 1 contours L185 L187 L190 L194 L195 | L199 L216 L219 L221 L230 | L184 L210 L218 L225 L228 | L188 L209 L211 L224 L255 bodies 1
extrude "Extrusion9" add sketch "Skizze1" along normal blind 3.7 contours A9 A30 A31 | A9 A30 | A16 A18 A23 | A16 A18 | A12 A25 | A12 A22 A25 | A10 A20 A26 | A10 A26 bodies 1
extrude "Extrusion10" add sketch "Skizze1" along normal blind 8.7 contours L231 L243 L253 L256 | L232 L249 L250 L260 | L248 L262 L270 L274 | L269 L272 L276 L323 | L271 L275 L316 L318 | L278 L281 L324 L340 | L291 L351 L352 L370 | L294 L297 L299 L305 | L301 L309 L320 L344 | L372 L392 L398 L402 | L373 L374 L399 L419 | L378 L418 L425 L437 | L379 L386 L393 L403 | L381 L385 L394 L448 | L404 L413 L434 L449 | L432 L438 L443 L451 bodies 1
combine "Kombinieren1" operation add target body 1 tool bodies 2
extrude "Extrusion11" add sketch "Skizze1" against normal blind 2.6 contours A4 | L98 L114 L133 L134 | A5 | A6 | A7 | L126 L128 L144 L155 | A8 | L132 L149 L377 | L132 L136 L149 L150 L377 L387 L408 L431 L444 | L132 L136 L408 L431 | L136 L150 L387 L444 | A9 A30 A31 | A9 L190 L193 L194 L197 L198 A28 A30 A31 | A9 L185 L187 L190 L193 L195 L197 L198 A28 | A16 L184 A18 L189 L196 A23 L198 L210 A29 | A16 L184 L189 L196 L198 L218 A29 L225 L228 | A12 L186 L191 L193 A24 L216 L219 L221 L230 | A12 L186 L191 L193 A22 A24 A25 L199 L219 | A16 A18 A23 | A12 A22 A25 | L185 L187 L190 L194 L195 | L199 L216 L219 L221 L230 | A10 A20 L188 L192 L196 A26 A27 L211 | A10 L188 L192 L196 A27 L209 L224 L255 | L184 L210 L218 L225 L228 | A10 A20 A26 | L188 L209 L211 L224 L255 | L135 L140 L143 L154 | L137 L138 L148 L151 | A11 | L142 L146 L147 L156 L384 L395 L397 L409 L410 | A13 | A14 | A15 | A17 | L231 L243 L253 L256 | L232 L249 L250 L260 | L248 L262 L270 L274 | L269 L272 L276 L323 | L271 L275 L316 L318 | L278 L281 L324 L340 | L291 L351 L352 L370 | L294 L297 L299 L305 | L301 L309 L320 L344 | L372 L392 L398 L402 | L373 L374 L399 L419 | L378 L418 L425 L437 | L379 L386 L393 L403 | L381 L385 L394 L448 | L404 L413 L434 L449 | L432 L438 L443 L451 bodies 1
fillet "Abrundung1" radius 0.5 4 edges at (9.1452, 26.1706, 5) (8.1452, 22.6706, 5) (9.1452, 19.1706, 5) (10.1452, 22.6706, 5) on bodies 1
ref_plane "Arbeitsebene2" through (0, 0, -10) normal (0, 0, 1) x (1, 0, 0)
sketch "Skizze4" plane through (0, 0, -10) normal (0, 0, 1) x (1, 0, 0)
  line L0 (1.2712, 50.8006) -> (57.1512, 50.8006)
  arc A0 (58.4212, 49.5306) -> (57.1512, 50.8006) centre (57.1512, 49.5306) ccw
  line L1 (58.4212, 49.5306) -> (58.4212, 0.7626)
  arc A1 (57.6592, 0.0006) -> (58.4212, 0.7626) centre (57.6592, 0.7626) ccw
  line L2 (57.6592, 0.0006) -> (0.7632, 0.0006)
  arc A2 (0.0012, 0.7626) -> (0.7632, 0.0006) centre (0.7632, 0.7626) ccw
  line L3 (0.0012, 0.7626) -> (0.0012, 49.5306)
  arc A3 (1.2712, 50.8006) -> (0.0012, 49.5306) centre (1.2712, 49.5306) ccw
  circle A4 centre (29.2112, 42.5006) radius 2.736
  line L4 (-2.0388, 56.8006) -> (60.4612, 56.8006)
  line L5 (63.4612, 53.8006) -> (63.4612, 0.0006)
  line L6 (63.4612, 0.0006) -> (-5.0388, 0.0006)
  line L7 (-5.0388, 0.0006) -> (-5.0388, 53.8006)
  arc A5 (-2.0388, 56.8006) -> (-5.0388, 53.8006) centre (-2.0388, 53.8006) ccw
  arc A6 (63.4612, 53.8006) -> (60.4612, 56.8006) centre (60.4612, 53.8006) ccw
  arc A7 (61.4612, 53.8006) -> (60.4612, 54.8006) centre (60.4612, 53.8006) ccw
  line L8 (-2.0388, 54.8006) -> (60.4612, 54.8006)
  arc A8 (-2.0388, 54.8006) -> (-3.0388, 53.8006) centre (-2.0388, 53.8006) ccw
  line L9 (-3.0388, 0.0006) -> (-3.0388, 53.8006)
  line L10 (61.4612, 53.8006) -> (61.4612, 0.0006)
  line L11 (-3.0388, 50.8006) -> (61.4612, 50.8006)
  line L12 (-3.0388, 48.8006) -> (61.4612, 48.8006)
  line L13 (-3.0388, 9.7006) -> (61.4612, 9.7006)
  line L14 (-3.0388, 11.7006) -> (61.4612, 11.7006)
  line L15 (0.0012, 48.8006) -> (0.0012, 11.7006)
  line L16 (58.4212, 48.8006) -> (58.4212, 11.7006)
  line L17 (2.0012, 48.8006) -> (2.0012, 11.7006)
  line L18 (56.4212, 48.8006) -> (56.4212, 11.7006)
  circle A9 centre (29.2112, 42.5006) radius 2.5
  circle A10 centre (29.2112, 42.5006) radius 1.25
  circle A11 centre (29.2112, 42.5006) radius 3.5
  line L19 (-0.2488, 11.7006) -> (-0.2488, 9.7006)
  line L20 (58.6712, 11.7006) -> (58.6712, 9.7006)
  arc A12 (-2.0388, 56.0006) -> (-4.2388, 53.8006) centre (-2.0388, 53.8006) ccw
  line L21 (-4.2388, 0.0006) -> (-4.2388, 53.8006)
  line L22 (62.6612, 53.8006) -> (62.6612, 0)
  arc A13 (62.6612, 53.8006) -> (60.4612, 56.0006) centre (60.4612, 53.8006) ccw
  line L23 (-2.0388, 56.0006) -> (60.4612, 56.0006)
  dimension "d41" = 68.5
  dimension "d42" = 6
  dimension "d43" = 3
  dimension "d44" = 3
  dimension "d46" = 2
  dimension "d47" = 2
  dimension "d48" = 9.7
  dimension "d49" = -2
  dimension "d50" = -2
  dimension "d51" = 2
  dimension "d52" = 5
  dimension "d53" = 2.5
  dimension "d54" = 7
  dimension "d55" = 0.25
  dimension "d56" = 0.25
  dimension "d58" = 0.8
  constraint horizontal L4
  constraint vertical L5
  constraint horizontal L6
  constraint vertical L7
  constraint midpoint L2 L6
  constraint tangent L4 A5
  constraint tangent L7 A5
  constraint tangent L4 A6
  constraint tangent L5 A6
  constraint concentric A6 A7
  constraint parallel L4 L8
  constraint concentric A5 A8
  constraint parallel L7 L9
  constraint parallel L5 L10
  constraint tangent A7 L10
  constraint tangent A7 L8
  constraint tangent L8 A8
  constraint tangent A8 L9
  constraint coincident L6 L9.start
  constraint coincident L6 L10.end
  constraint coincident L9 L11.start
  constraint coincident L10 L11.end
  constraint perpendicular L10 L11
  constraint collinear L0 L11
  constraint coincident L9 L13.start
  constraint coincident L10 L13.end
  constraint perpendicular L10 L13
  constraint coincident L12 L15.start
  constraint coincident L3 L15.start
  constraint coincident L14 L15.end
  constraint coincident L3 L15.end
  constraint coincident L1 L16.start
  constraint coincident L12 L16.start
  constraint coincident L14 L16.end
  constraint coincident L1 L16.end
  constraint concentric A4 A9
  constraint concentric A9 A10
  constraint concentric A10 A11
  constraint coincident L14 L19.start
  constraint coincident L13 L19.end
  constraint perpendicular L13 L19
  constraint coincident L14 L20.start
  constraint coincident L13 L20.end
  constraint perpendicular L13 L20
  constraint concentric A5 A12
  constraint parallel L7 L21
  constraint parallel L5 L22
  constraint concentric A6 A13
  constraint parallel L4 L23
  constraint tangent A13 L23
  constraint tangent A12 L23
  constraint tangent A12 L21
  constraint tangent L22 A13
  constraint coincident L6 L21.start
  measures "d41" distance of L5.end L6.end
  measures "d42" distance of L0 L4
  measures "d43" radius of A5
  measures "d44" radius of A6
  measures "d46" distance of L4 L8
  measures "d48" distance of L10.end L13.end
  measures "d52" diameter of A9
  measures "d53" diameter of A10
  measures "d54" diameter of A11
  measures "d55" distance of L3 L19
  measures "d56" distance of L1 L20
  measures "d58" distance of L5 L22
extrude "Extrusion12" add sketch "Skizze4" along normal blind 2 separate body contours L0 A7 L8 A8 L9 L10 L11 | L0 A0 L1 L3 A3 L11 L12 | L3 A3 L9 L11 L12 | A0 L1 L10 L11 L12 | L6 A7 L8 A8 L9 L10 A12 L21 L22 A13 L23 | L3 L12 L14 L15 L17 | L3 L9 L12 L14 L15 | L1 L10 L12 L14 L16 | L1 L12 L14 L16 L18 | L1 L3 L13 L14 | L3 L13 L14 L19 | L12 L14 L17 L18 | L9 L13 L14 L19 | L1 L13 L14 L20 | L10 L13 L14 L20 | L1 A1 L2 A2 L3 L6 L13 | A2 L3 L6 L9 L13 | L1 A1 L6 L10 L13 | L4 L5 L6 L7 A5 A6 A12 L21 L22 A13 L23 | A4 | A9 | A10 | A11 makes body 3
extrude "Extrusion14" add sketch "Skizze4" along normal blind 8.4 contours L0 A0 L1 L3 A3 L11 L12 | L3 A3 L9 L11 L12 | A0 L1 L10 L11 L12 | L3 L12 L14 L15 L17 | L1 L12 L14 L16 L18 | L1 L3 L13 L14 | L3 L13 L14 L19 | L1 L13 L14 L20 | A4 | A11 bodies 3
extrude "Extrusion15" add sketch "Skizze4" along normal blind 8.4 contours L6 A7 L8 A8 L9 L10 A12 L21 L22 A13 L23 bodies 3
extrude "Extrusion16" add sketch "Skizze4" along normal blind 10 contours L9 L13 L14 L19 | L10 L13 L14 L20 | L4 L5 L6 L7 A5 A6 A12 L21 L22 A13 L23 | A9 bodies 3
fillet "Abrundung2" radius 3 5 edges at (-5.0388, 26.9006, -10) (-4.1602, 55.9219, -10) (29.2112, 56.8006, -10) (62.5825, 55.9219, -10) (63.4612, 26.9006, -10) on bodies 3
fillet "Abrundung3" radius 1 4 edges at (29.2112, 48.8006, -8) (56.4212, 30.2506, -8) (2.0012, 30.2506, -8) (29.2112, 11.7006, -8) on bodies 3
fillet "Abrundung4" radius 1 6 edges at (29.2112, 50.8006, -8) (61.4612, 52.3006, -8) (61.1683, 54.5077, -8) (29.2112, 54.8006, -8) (-2.746, 54.5077, -8) (-3.0388, 52.3006, -8) on bodies 3
fillet "Abrundung5" radius 1 1 edges at (25.948, 43.7663, -8) on bodies 3
fillet "Abrundung6" radius 1 4 edges at (-3.0388, 30.2506, -8) (-1.5188, 48.8006, -8) (-1.5188, 11.7006, -8) (0.0012, 30.2506, -8) on bodies 3
fillet "Abrundung7" radius 1 4 edges at (58.4212, 30.2506, -8) (59.9412, 48.8006, -8) (59.9412, 11.7006, -8) (61.4612, 30.2506, -8) on bodies 3
fillet "Abrundung8" radius 1 3 edges at (-3.0388, 4.8506, -8) (29.2112, 9.7006, -8) (61.4612, 4.8506, -8) on bodies 3
ref_plane "Arbeitsebene4" through (29.2112, 25.4006, 12) normal (0, 0, 1) x (1, 0, 0)